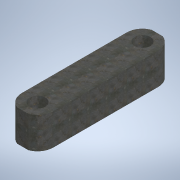
# Autodesk Inventor part: Middle v2
Saved by Autodesk Inventor 2021 (Build 250183000, 183)
## iProperties
Created: 2022-04-30
Part Number: Middle v2
Material: Steel
Document SubType Name: Sheet Metal
Designer: youss
Density: 7.85 g/cm^3
Sheet Metal Rule: Default_mm
Appearance: Plate
Author: youss
Autodesk Inventor part; units mm, degrees
ref_plane "YZ Plane" through (0, 0, 0) normal (1, 0, 0) x (0, 1, 0)
ref_plane "XZ Plane" through (0, 0, 0) normal (0, 1, 0) x (-1, 0, 0)
ref_plane "XY Plane" through (0, 0, 0) normal (0, 0, 1) x (1, 0, 0)
sketch "Sketch1" plane through (0, 0, 0) normal (0, 1, 0) x (-1, 0, 0)
  line L0 (0, 0) -> (0, -1000)
  line L1 (0, -1000) -> (150, -1000)
  line L2 (150, -1000) -> (150, 0)
  circle A0 centre (150, 0) radius 150
  circle A1 centre (150, -1000) radius 150
  line L3 (300, 0) -> (300, -1000)
  circle A2 centre (150, 0) radius 75
  circle A3 centre (150, -1000) radius 75
  dimension "d0" = 1000
  dimension "d1" = 150
  dimension "d2" = 1000
  dimension "d3" = 150
  dimension "d4" = 150
  constraints: 8 end point, 4 centre point, 4 coincident, 4 point on circle, 2 vertical, 1 perpendicular, 1 tangent
  measures "d0" distance of L0.start L0.end
  measures "d1" distance of L0.end L1.end
  measures "d2" distance of L1.end L2.end
  measures "d3" diameter of A2
  measures "d4" diameter of A3
extrude "Extrusion1" add sketch "Sketch1" along normal blind 300 contours A0 L2 A1 L0 | A0 | A1 L2 A3 L1 | L1 A3 L2 A1 | L3 A1 L2 A0
sketch "Sketch2" plane through (0, 0, 0) normal (0, -1, 0) x (1, 0, 0)
  line L0 (0, 0) -> (-300, 0)
  line L1 (0, 140) -> (-300, 140)
  circle A0 centre (-150, 0) radius 150
  circle A1 centre (-150, -1000) radius 75 projected
  circle A2 centre (-150, -1000) radius 150
  arc A3 (-300, -1000) -> (0, -1000) centre (-150, -1000) ccw projected
  line L2 (-300, -1000) -> (0, -1000)
  line L3 (-300, -1140) -> (0, -1140)
  point P0 (-96.1484, -1140)
  point P1 (-203.8516, -1140)
  point P2 (-203.8516, 140)
  point P3 (-96.1484, 140)
  dimension "d7" = 140
  dimension "d8" = 140
  constraints: 8 end point, 2 centre point, 2 horizontal, 2 parallel, 1 coincident, 1 midpoint
  measures "d7" distance between parallel lines of L0 L1
  measures "d8" distance between parallel lines of L2 L3
extrude "Extrusion2" cut sketch "Sketch2" against normal through all contours L1 A0 | A2 L3
equation "\"BendRadius\" = Thickness"
equation "\"BendReliefWidth\" = Thickness"
equation "\"BendReliefDepth\" = 0.5 * Thickness"
equation "\"CornerReliefSize\" = 4 * Thickness"
equation "\"MinimumRemnant\" = 2 * Thickness"
equation "\"TransitionRadius\" = BendRadius"
equation "\"JacobiRadiusSize\" = BendRadius"
equation "\"GapSize\" = Thickness"
equation "\"Thickness\" = 0.5"
body "Solid1"
